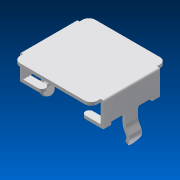
# Autodesk Inventor part: 12mm Incremental Encoder Anti-Rotation Plate
Saved by Autodesk Inventor 2014 (Build 180170000, 170)
## iProperties
Created: 2011-11-07
Part Number: 12mm Incremental Encoder Anti-Rotation Plate
Document SubType Name: Modeling
Designer: sdarley
Density: 1 g/cm^3
Material: Generic
Appearance: Polished Brushed
Author: sdarley
Autodesk Inventor part; units mm, degrees
ref_plane "YZ Plane" through (0, 0, 0) normal (1, 0, 0) x (0, 1, 0)
ref_plane "XZ Plane" through (0, 0, 0) normal (0, 1, 0) x (-1, 0, 0)
ref_plane "XY Plane" through (0, 0, 0) normal (0, 0, 1) x (1, 0, 0)
sketch "Sketch1" plane through (0, 0, 0) normal (0, 0, 1) x (1, 0, 0)
  arc A0 (6.175, 5) -> (5.175, 6) centre (5.175, 5) ccw projected
  line L0 (-5.175, 6) -> (5.175, 6) projected
  arc A1 (-5.175, 6) -> (-6.175, 5) centre (-5.175, 5) ccw projected
  line L1 (-6.175, -5) -> (-6.175, 5) projected
  arc A2 (-6.175, -5) -> (-5.175, -6) centre (-5.175, -5) ccw projected
  line L2 (5.175, -6) -> (-5.175, -6) projected
  arc A3 (5.175, -6) -> (6.175, -5) centre (5.175, -5) ccw projected
  line L3 (6.175, 5) -> (6.175, -5) projected
  line L4 (-6.175, 4.5) -> (-6.675, 4.5)
  line L5 (-6.675, 4.5) -> (-6.675, -4.5)
  line L6 (-6.675, -4.5) -> (-6.175, -4.5)
  line L7 (-6.175, -4.5) -> (-6.175, 4.5)
  line L8 (6.175, 4.5) -> (6.675, 4.5)
  line L9 (6.675, 4.5) -> (6.675, -4.5)
  line L10 (6.675, -4.5) -> (6.175, -4.5)
  line L11 (6.175, -4.5) -> (6.175, 4.5)
  point P0 (0, 0)
  point P1 (-6.175, 0)
  point P2 (-6.175, 0)
  point P3 (6.175, 0)
  point P4 (6.175, 0)
  dimension "d0" = 0.5
  dimension "d1" = 9
  dimension "d2" = 0.5
  dimension "d3" = 9
  constraints: 16 end point, 4 midpoint, 4 parallel, 2 coincident, 2 horizontal, 2 perpendicular, 2 point on line
  measures "d0" distance of L6.end L5.end
  measures "d1" distance of L5.end L4.end
  measures "d2" distance of L9.end L10.end
  measures "d3" distance between parallel lines of L8 L10
extrude "Extrusion1" add sketch "Sketch1" along normal blind 0.5
sketch "Sketch2" plane through (0, 0, 0) normal (0, 0, -1) x (-1, 0, 0)
  line L0 (-6.675, 4.5) -> (-6.175, 4.5) projected
  line L1 (-6.675, -4.5) -> (-6.675, 4.5) projected
  line L2 (-6.175, -4.5) -> (-6.675, -4.5) projected
  line L3 (-6.175, -5) -> (-6.175, -4.5) projected
  arc A0 (-6.175, -5) -> (-5.175, -6) centre (-5.175, -5) ccw projected
  line L4 (5.175, -6) -> (-5.175, -6) projected
  arc A1 (5.175, -6) -> (6.175, -5) centre (5.175, -5) ccw projected
  line L5 (6.175, -4.5) -> (6.175, -5) projected
  line L6 (6.675, -4.5) -> (6.175, -4.5) projected
  line L7 (6.675, 4.5) -> (6.675, -4.5) projected
  line L8 (6.175, 4.5) -> (6.675, 4.5) projected
  line L9 (6.175, 5) -> (6.175, 4.5) projected
  arc A2 (6.175, 5) -> (5.175, 6) centre (5.175, 5) ccw projected
  line L10 (-5.175, 6) -> (5.175, 6) projected
  arc A3 (-5.175, 6) -> (-6.175, 5) centre (-5.175, 5) ccw projected
  line L11 (-6.175, 4.5) -> (-6.175, 5) projected
  line L12 (6.075, 5) -> (6.075, 4.6) projected
  arc A4 (6.075, 5) -> (5.175, 5.9) centre (5.175, 5) ccw projected
  line L13 (-5.175, 5.9) -> (5.175, 5.9) projected
  arc A5 (-5.175, 5.9) -> (-6.075, 5) centre (-5.175, 5) ccw projected
  line L14 (-6.075, 4.6) -> (-6.075, 5) projected
  line L15 (6.075, 4.6) -> (-6.075, 4.6) projected
  line L16 (-6.175, 5) -> (-6.175, -5) projected
  line L17 (6.175, -5) -> (6.175, 5) projected
  point P0 (0, 0)
extrude "Extrusion4" add sketch "Sketch2" along normal blind 3 contours L0 L16 L2 L1 | L8 L7 L6 L17
sketch "Sketch3" plane through (0, 0, -3) normal (0, 0, -1) x (-1, 0, 0)
  line L0 (-6.175, -4.5) -> (-6.175, 4.5)
  line L1 (-6.675, -4.5) -> (-6.675, 4.5)
  line L2 (6.175, 4.5) -> (6.175, -4.5)
  line L3 (6.675, -4.5) -> (6.175, -4.5)
  line L4 (6.675, 4.5) -> (6.675, -4.5)
  line L5 (6.175, 4.5) -> (6.675, 4.5)
  line L6 (-6.675, 1) -> (-6.175, 1)
  line L7 (-6.175, 1) -> (-6.175, -1)
  line L8 (-6.175, -1) -> (-6.675, -1)
  line L9 (-6.675, -1) -> (-6.675, 1)
  line L10 (6.175, 1) -> (6.675, 1)
  line L11 (6.675, 1) -> (6.675, -1)
  line L12 (6.675, -1) -> (6.175, -1)
  line L13 (6.175, -1) -> (6.175, 1)
  line L14 (-6.175, -4.5) -> (-6.175, 4.5) projected
  line L15 (-6.675, 4.5) -> (-6.175, 4.5) projected
  line L16 (-6.675, -4.5) -> (-6.675, 4.5) projected
  line L17 (-6.175, -4.5) -> (-6.675, -4.5) projected
  point P0 (0, 0)
  point P1 (-6.675, 0)
  point P2 (-6.675, 0)
  point P3 (6.675, 0)
  point P4 (6.675, 0)
  dimension "d8" = 2
  dimension "d9" = 2
  constraints: 28 end point, 4 midpoint, 4 parallel, 4 point on line, 2 coincident, 2 horizontal, 2 perpendicular
  measures "d8" distance between parallel lines of L12 L10
  measures "d9" distance between parallel lines of L8 L6
extrude "Extrusion3" add sketch "Sketch3" along normal blind 2 contours L8 L1 L6 L0 | L10 L4 L12 L2
sketch "Sketch7" plane through (-6.675, -1, -3) normal (0, -1, 0) x (1, 0, 0)
  line L0 (0.5, 0) -> (0.5, -2) projected
  line L1 (0, 0) -> (0, -2) projected
  line L2 (12.85, -2) -> (13.35, -2) projected
  line L3 (13.35, 0) -> (13.35, -2) projected
  line L4 (12.85, 0) -> (13.35, 0) projected
  line L5 (12.85, 0) -> (12.85, -2) projected
  line L6 (0.183, -2.5776) -> (-0.0465, -2.9752)
  line L7 (0.5, -2) -> (2, -2) construction
  line L8 (0.4495, -4.4856) -> (0.0165, -4.7356)
  line L9 (0.0165, -4.7356) -> (-0.4835, -3.8696)
  line L10 (-0.0313, -3.653) -> (0.4495, -4.4856)
  line L11 (0, -1.3946) -> (0.5, -1.3946)
  line L12 (0.5, -1.3946) -> (0.5, -1.4408)
  arc A0 (-0.25, -2.3276) -> (0, -1.3946) centre (-1.6937, -1.4408) ccw
  arc A1 (0.183, -2.5776) -> (0.5, -1.3946) centre (-1.866, -1.3946) ccw
  arc A2 (-0.0147, -2.9201) -> (-0.0313, -3.653) centre (0.5799, -3.3001) ccw
  arc A3 (-0.4835, -2.7321) -> (-0.4835, -3.8696) centre (0.5016, -3.3008) ccw
  line L13 (-0.4835, -2.7321) -> (-0.2038, -2.2476)
  line L14 (0.4773, -1.0678) -> (0.5, -1.0286)
  line L15 (0, 0) -> (0.5, 0) projected
  line L16 (6.675, 3) -> (6.675, -7.5031) construction
  line L17 (13.167, -2.5776) -> (13.3965, -2.9752)
  line L18 (12.9005, -4.4856) -> (13.3335, -4.7356)
  line L19 (13.3335, -4.7356) -> (13.8335, -3.8696)
  line L20 (13.3813, -3.653) -> (12.9005, -4.4856)
  line L21 (13.35, -1.3946) -> (12.85, -1.3946)
  arc A4 (13.35, -1.3946) -> (13.6, -2.3276) centre (15.0437, -1.4408) ccw
  arc A5 (12.85, -1.3946) -> (13.167, -2.5776) centre (15.216, -1.3946) ccw
  arc A6 (13.3813, -3.653) -> (13.3647, -2.9201) centre (12.7701, -3.3001) ccw
  arc A7 (13.8335, -3.8696) -> (13.8335, -2.7321) centre (12.8484, -3.3008) ccw
  line L22 (13.8335, -2.7321) -> (13.5538, -2.2476)
  point P0 (0.1706, -2.597)
  point P1 (-0.4453, -2.6697)
  point P2 (-0.0137, -2.9183)
  dimension "d40" = 120
  dimension "d57" = 0.5
  dimension "d58" = 0.5
  dimension "d59" = 1
  constraints: 32 end point, 21 point on circle, 16 symmetric about line, 8 centre point, 8 point on line, 5 perpendicular, 4 tangent, 2 parallel, 1 horizontal, 4 other
  measures "d40" angle of L6 L7
  measures "d57" distance between parallel lines of L9 L10
  measures "d58" distance between parallel lines of L6 L13
  measures "d59" distance of L8.end L9.end
extrude "Extrusion8" add sketch "Sketch7" against normal blind 2 contours L0 A1 L6 A2 L10 L8 L9 A3 L13 A0 L11 | A4 L22 A7 L19 L18 L20 A6 L17 A5 L2 L3 | A5 L21 L3 L2
sketch "Sketch8" plane through (-6.675, -1, -3) normal (0, -1, 0) x (1, 0, 0)
  line L0 (-0.0147, -2.9201) -> (0.183, -2.5776) projected
  arc A0 (0.183, -2.5776) -> (0.4212, -2) centre (-1.866, -1.3946) ccw projected
  line L1 (0.4212, -2) -> (0.5, -2) projected
  line L2 (0.5, 0) -> (0.5, -2) projected
  arc A1 (0.4212, -2) -> (0.5, -1.3946) centre (-1.866, -1.3946) ccw
  line L3 (0.5, -1.3946) -> (0.5, -2)
  line L4 (0, 0) -> (0.5, 0) projected
  line L5 (6.675, 3) -> (6.675, -5.8732) construction
  line L6 (12.9288, -2) -> (12.85, -2)
  line L7 (12.85, 0) -> (12.85, -2)
  arc A2 (12.85, -1.3946) -> (12.9288, -2) centre (15.216, -1.3946) ccw
  constraints: 8 end point, 6 symmetric about line, 4 point on circle, 4 point on line, 3 tangent, 2 centre point, 1 coincident, 1 collinear, 1 perpendicular, 1 other
extrude "Extrusion9" cut sketch "Sketch8" against normal through all
fillet "Fillet1" radius 0.25 6 edges at (6.425, 1, -3) (6.425, -1, -3) (-6.425, 1, -3) (-6.425, -1, -3) (-6.675, 0, 0.5) (6.675, 0, 0.5)
sketch "Sketch4" plane through (0, 0, -3) normal (0, 0, -1) x (-1, 0, 0)
  line L0 (-6.675, -4.5) -> (-6.675, -1.25) projected
  line L1 (-6.175, -4.5) -> (-6.675, -4.5) projected
  line L2 (-6.175, -4.5) -> (-6.175, -1.25) projected
  line L3 (-6.175, 1.25) -> (-6.675, 1.25) projected
  line L4 (-6.175, 1.25) -> (-6.175, 4.5) projected
  line L5 (-6.675, 4.5) -> (-6.175, 4.5) projected
  line L6 (-6.675, 1.25) -> (-6.675, 4.5) projected
  line L7 (6.675, 1.25) -> (6.175, 1.25) projected
  line L8 (6.675, 4.5) -> (6.675, 1.25) projected
  line L9 (6.175, 4.5) -> (6.675, 4.5) projected
  line L10 (6.175, 4.5) -> (6.175, 1.25) projected
  line L11 (6.175, -1.25) -> (6.675, -1.25) projected
  line L12 (6.175, -1.25) -> (6.175, -4.5) projected
  line L13 (6.675, -4.5) -> (6.175, -4.5) projected
  line L14 (6.675, -1.25) -> (6.675, -4.5) projected
  line L15 (-6.175, -3.3) -> (-6.675, -3.3)
  line L16 (-6.675, -3.3) -> (-6.675, -4.5)
  line L17 (-6.675, -4.5) -> (-6.175, -4.5)
  line L18 (-6.175, -4.5) -> (-6.175, -3.3)
  line L19 (-6.675, 4.5) -> (-6.175, 4.5)
  line L20 (-6.175, 4.5) -> (-6.175, 3.3)
  line L21 (-6.175, 3.3) -> (-6.675, 3.3)
  line L22 (-6.675, 3.3) -> (-6.675, 4.5)
  line L23 (6.175, 4.5) -> (6.675, 4.5)
  line L24 (6.675, 4.5) -> (6.675, 3.3)
  line L25 (6.675, 3.3) -> (6.175, 3.3)
  line L26 (6.175, 3.3) -> (6.175, 4.5)
  line L27 (6.175, -3.3) -> (6.675, -3.3)
  line L28 (6.675, -3.3) -> (6.675, -4.5)
  line L29 (6.675, -4.5) -> (6.175, -4.5)
  line L30 (6.175, -4.5) -> (6.175, -3.3)
  point P0 (0, 0)
  dimension "d17" = 1.2
  dimension "d18" = 0
  dimension "d19" = 1.2
  dimension "d20" = 0
  dimension "d21" = 1.2
  dimension "d22" = 1.2
  dimension "d23" = 0
  dimension "d24" = 0
  constraints: 32 end point, 8 parallel, 8 point on line, 4 horizontal, 4 perpendicular
  measures "d17" distance of L16.end L15.end
  measures "d18" distance between parallel lines of L1 L17
  measures "d19" distance of L19.end L20.end
  measures "d20" distance between parallel lines of L5 L19
  measures "d21" distance between parallel lines of L29 L27
  measures "d22" distance between parallel lines of L23 L25
  measures "d23" distance between parallel lines of L9 L23
  measures "d24" distance between parallel lines of L13 L29
extrude "Extrusion5" add sketch "Sketch4" along normal blind 0.5 contours L0 L15 L2 L1 | L21 L6 L5 L4 | L25 L10 L9 L8 | L27 L14 L13 L12
sketch "Sketch5" plane through (-6.175, -4.5, 0) normal (1, 0, 0) x (0, 0, -1)
  line L0 (3, 7.8) -> (3.5, 7.8) projected
  line L1 (3.5, 7.8) -> (3.5, 9) projected
  line L2 (0, 9) -> (3.5, 9) projected
  line L3 (0, 0) -> (3.5, 0) projected
  line L4 (3.5, 0) -> (3.5, 1.2) projected
  line L5 (3, 1.2) -> (3.5, 1.2) projected
  line L6 (3.25, 3.5) -> (4.3946, 3.5) projected
  line L7 (3, 0) -> (3, 1.2)
  line L8 (3, 7.8) -> (3, 9)
  point P0 (7, 3.5)
  point P1 (0, 4.5)
  constraints: 4 end point, 3 point on line, 1 collinear, 1 perpendicular
extrude "Extrusion6" add sketch "Sketch5" along normal blind 3
fillet "Fillet4" radius 0.1 4 edges at (-6.175, -3.9, -3) (-6.675, -3.9, -3.5) (-6.675, 3.9, -3.5) (-6.175, 3.9, -3)
fillet "Fillet5" radius 0.6 4 edges at (-3.175, -4.5, -3.25) (-3.175, -3.3, -3.25) (-3.175, 3.3, -3.25) (-3.175, 4.5, -3.25)
sketch "Sketch6" plane through (6.175, -4.5, 0) normal (-1, 0, 0) x (0, 0, 1)
  line L0 (-3, 1.2) -> (-3.5, 1.2) projected
  line L1 (-3.5, 1.2) -> (-3.5, 0) projected
  line L2 (0, 0) -> (-3.5, 0) projected
  line L3 (0, 9) -> (-3.5, 9) projected
  line L4 (-3.5, 9) -> (-3.5, 7.8) projected
  line L5 (-3, 7.8) -> (-3.5, 7.8) projected
  line L6 (-3, 7.8) -> (-3, 9)
  line L7 (-3, 1.2) -> (-3, 0)
  point P0 (0, 4.5)
  constraints: 4 end point, 2 perpendicular, 2 point on line
extrude "Extrusion7" add sketch "Sketch6" along normal blind 3
fillet "Fillet6" radius 0.1 4 edges at (6.675, 3.9, -3.5) (6.175, 3.9, -3) (6.675, -3.9, -3.5) (6.175, -3.9, -3)
fillet "Fillet7" radius 0.6 4 edges at (3.175, 4.5, -3.25) (3.175, 3.3, -3.25) (3.175, -3.3, -3.25) (3.175, -4.5, -3.25)
fillet "Fillet8" radius 1 4 edges at (-6.442, -1, -7.6106) (-6.442, 1, -7.6106) (6.442, -1, -7.6106) (6.442, 1, -7.6106)
equation "\"d3\" = d1"
equation "\"d9\" = d8"
equation "\"d58\" = d57"
equation "\"d19\" = d17"
equation "\"d21\" = d17"
equation "\"d22\" = d17"
body "Solid1"
